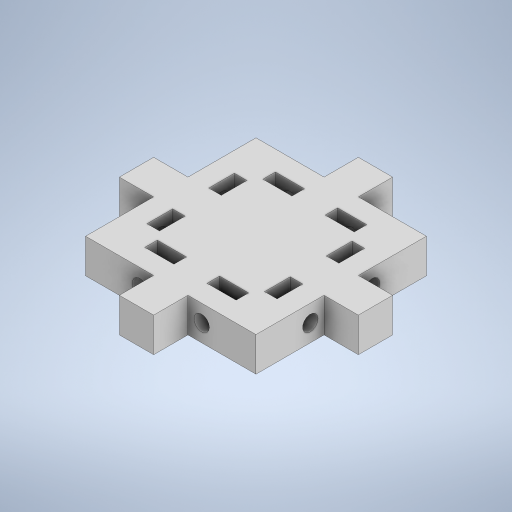
# Autodesk Inventor part: arm_motor_connect
Saved by Autodesk Inventor 2024 (Build 280153000, 153)
## iProperties
Created: 2024-09-18
Part Number: arm_motor_connect
Material: 일반
Document SubType Name: Modeling
Designer: Eungang
Density: 1 g/cm^3
Appearance: 기본값
Author: Eungang
Autodesk Inventor part; units mm, degrees
ref_plane "YZ Plane" through (0, 0, 0) normal (1, 0, 0) x (0, 1, 0)
ref_plane "XZ Plane" through (0, 0, 0) normal (0, 1, 0) x (-1, 0, 0)
sketch "스케치1" plane through (0, 0, 0) normal (0, 0, 1) x (1, 0, 0)
  arc A0 (-4.555, 20.4) -> (-1.5118, 17.2038) centre (-1.355, 20.4) ccw projected
  line L0 (-4.555, 20.4) -> (-4.555, 29.4) projected
  line L1 (-4.555, 29.4) -> (-9.955, 29.4) projected
  line L2 (-9.955, 29.4) -> (-9.955, 17.8) projected
  line L3 (-9.955, 17.8) -> (-4.855, 11.8) projected
  line L4 (-4.855, 11.8) -> (-4.7625, 11.8) projected
  line L5 (-4.7625, 11.8) -> (-4.7625, -3) projected
  line L6 (-4.7625, -3) -> (3.7037, -3) projected
  arc A1 (4.7037, -2) -> (3.7037, -3) centre (4.7037, -3) ccw projected
  line L7 (4.7037, -2) -> (4.7037, 2.1) projected
  arc A2 (5.6987, 3) -> (4.7037, 2.1) centre (4.7037, 3.1) ccw projected
  line L8 (5.6987, 3) -> (9.9088, 3) projected
  arc A3 (10.9037, 2.1) -> (9.9088, 3) centre (10.9037, 3.1) ccw projected
  line L9 (10.9037, 2.1) -> (10.9037, -2) projected
  arc A4 (11.9037, -3) -> (10.9037, -2) centre (10.9037, -3) ccw projected
  line L10 (11.9037, -3) -> (20.4525, -3) projected
  line L11 (20.4525, -3) -> (20.4525, 11.8) projected
  line L12 (20.4525, 11.8) -> (20.545, 11.8) projected
  line L13 (20.545, 11.8) -> (25.645, 17.8) projected
  line L14 (25.645, 17.8) -> (25.645, 29.4) projected
  line L15 (25.645, 29.4) -> (20.245, 29.4) projected
  line L16 (20.245, 29.4) -> (20.245, 20.4) projected
  arc A5 (17.2018, 17.2038) -> (20.245, 20.4) centre (17.045, 20.4) ccw projected
  line L17 (17.2018, 17.2038) -> (-1.5118, 17.2038) projected
  circle A6 centre (13.2469, 0) radius 1.35 projected
  circle A7 centre (2.4432, 0) radius 1.35 projected
  circle A8 centre (18.0506, 0) radius 1.35 projected
  circle A9 centre (-2.3606, 0) radius 1.35 projected
  circle A10 centre (-7.155, 20.9) radius 1.35 projected
  circle A11 centre (-0.655, 14.6) radius 1.35 projected
  circle A12 centre (16.345, 14.6) radius 1.35 projected
  circle A13 centre (22.845, 20.9) radius 1.35 projected
  line L18 (20.4525, -3) -> (-4.855, -3)
  line L19 (-4.855, -3) -> (-4.855, 3)
  line L20 (-4.855, 3) -> (20.4525, 3)
  line L21 (20.4525, 3) -> (20.4525, -3)
  line L22 (22.845, 3) -> (22.845, -11.8) projected
  line L23 (-7.155, 3) -> (-7.155, -11.8) projected
  line L24 (22.745, 3) -> (22.745, -11.8)
  line L25 (-7.055, 3) -> (-7.055, -11.8)
  line L26 (22.745, -3) -> (-7.055, -3)
  line L27 (-7.055, -3) -> (-7.055, 3)
  line L28 (-7.055, 3) -> (22.745, 3)
  line L29 (22.745, 3) -> (22.745, -3)
  point P0 (0, 0)
  point P1 (11.8625, -3)
  point P2 (20.4525, 3)
  point P3 (9.8675, 3)
  point P4 (5.6574, 3)
  point P5 (-4.7625, 3)
  point P6 (3.6625, -3)
  point P7 (-4.855, 3)
  point P8 (-7.055, -3)
  point P9 (-4.855, -3)
  point P10 (-4.7625, -3)
  point P11 (22.745, 1.2049)
  point P12 (20.4525, 3)
  point P13 (20.4525, -3)
  point P14 (11.8987, 3)
  point P15 (3.7037, -3)
  point P16 (11.9037, -3)
  point P17 (5.6987, 3)
  point P18 (3.7088, 3)
  point P19 (5.6987, 3)
  point P20 (11.9037, -3)
  point P21 (-4.7625, 3)
  point P22 (-4.855, -3)
  point P23 (10.9037, -1.792)
  point P24 (-4.7625, -3)
  point P25 (4.7037, -1.792)
  dimension "d7" = 0.1
  dimension "d8" = 0.1
  constraints: 20 end point, 6 parallel, 2 horizontal, 2 perpendicular, 1 point on line
  measures "d7" distance between parallel lines of L22 L24
  measures "d8" distance between parallel lines of L23 L25
extrude "돌출1" add sketch "스케치1" along normal blind 29.8 contours L20 A2 L7 A1 L6 L5 | L5 L18 L19 L20 | L19 L26 L25 L28 | L20 L8 A3 L9 A4 L18 A1 L7 A2 | L28 L24 L26 L11 | L11 L10 A4 L9 A3 L20 | A6 | A7 | A8 | A9
ref_plane "작업 평면4" through (10.8037, 3, 0) normal (0, 1, 0) x (1, 0, 0)
sketch "스케치5" plane through (10.8037, 3, 0) normal (0, 1, 0) x (1, 0, 0)
  line L0 (1.1931, -3.675) -> (1.1931, 6)
  line L1 (3.6931, -3.675) -> (3.6931, 6)
  line L2 (1.1931, -5.675) -> (3.6931, -5.675)
  line L3 (2.4431, 0) -> (2.4431, -3.675)
  line L4 (2.4431, -5.675) -> (2.4431, -4.575)
  line L5 (2.4431, -4.575) -> (2.4431, -3.475)
  line L6 (2.4431, -3.475) -> (-0.1069, -3.475)
  line L7 (2.4431, -3.475) -> (4.9931, -3.475)
  line L8 (4.9931, -3.475) -> (-0.1069, -3.475)
  line L9 (-0.1069, -3.475) -> (-0.1069, -5.675)
  line L10 (-0.1069, -5.675) -> (4.9931, -5.675)
  line L11 (4.9931, -5.675) -> (4.9931, -3.475)
  line L12 (1.1931, -5.675) -> (1.1931, 6)
  line L13 (3.6931, -5.675) -> (3.6931, 6)
  line L14 (1.1931, -5.675) -> (3.6931, -5.675)
  line L15 (2.4431, -3.675) -> (2.4431, -5.675)
  line L16 (-23.9, -14.9) -> (17.9, -14.9)
  line L17 (1.1931, -24.125) -> (3.6931, -24.125)
  line L18 (2.4431, -24.125) -> (2.4431, -25.225)
  line L19 (2.4431, -25.225) -> (2.4431, -26.325)
  line L20 (2.4431, -26.325) -> (-0.1069, -26.325)
  line L21 (2.4431, -26.325) -> (4.9931, -26.325)
  line L22 (4.9931, -26.325) -> (-0.1069, -26.325)
  line L23 (-0.1069, -26.325) -> (-0.1069, -24.125)
  line L24 (-0.1069, -24.125) -> (4.9931, -24.125)
  line L25 (4.9931, -24.125) -> (4.9931, -26.325)
  line L26 (1.1931, -24.125) -> (3.6931, -24.125)
  line L27 (2.4431, -26.125) -> (2.4431, -24.125)
  line L28 (-3, -14.9) -> (-3, -22)
  line L29 (-7.1931, -5.675) -> (-9.6931, -5.675)
  line L30 (-8.4431, -5.675) -> (-8.4431, -4.575)
  line L31 (-8.4431, -4.575) -> (-8.4431, -3.475)
  line L32 (-8.4431, -3.475) -> (-5.8931, -3.475)
  line L33 (-8.4431, -3.475) -> (-10.9931, -3.475)
  line L34 (-10.9931, -3.475) -> (-5.8931, -3.475)
  line L35 (-5.8931, -3.475) -> (-5.8931, -5.675)
  line L36 (-5.8931, -5.675) -> (-10.9931, -5.675)
  line L37 (-10.9931, -5.675) -> (-10.9931, -3.475)
  line L38 (-7.1931, -5.675) -> (-9.6931, -5.675)
  line L39 (-8.4431, -3.675) -> (-8.4431, -5.675)
  line L40 (-7.1931, -24.125) -> (-9.6931, -24.125)
  line L41 (-8.4431, -24.125) -> (-8.4431, -25.225)
  line L42 (-8.4431, -25.225) -> (-8.4431, -26.325)
  line L43 (-7.1931, -24.125) -> (-9.6931, -24.125)
  line L44 (-8.4431, -26.125) -> (-8.4431, -24.125)
  line L45 (-8.4431, -26.325) -> (-10.9931, -26.325)
  line L46 (-10.9931, -24.125) -> (-10.9931, -26.325)
  line L47 (-8.4431, -26.325) -> (-5.8931, -26.325)
  line L48 (-5.8931, -26.325) -> (-5.8931, -24.125)
  line L49 (-10.9931, -26.325) -> (-5.8931, -26.325)
  line L50 (-5.8931, -24.125) -> (-10.9931, -24.125)
  line L51 (-12.1837, -21.5519) -> (-23.8587, -21.5519)
  line L52 (-12.1837, -19.0519) -> (-23.8587, -19.0519)
  line L53 (-12.1837, -19.0519) -> (-12.1837, -21.5519)
  line L54 (-12.1837, -19.0519) -> (-14.3837, -19.0519)
  line L55 (-12.1837, -20.3019) -> (-12.1837, -18.0519)
  line L56 (-12.1837, -20.3019) -> (-12.1837, -22.5519)
  line L57 (-14.3837, -18.0519) -> (-12.1837, -18.0519)
  line L58 (-12.1837, -18.0519) -> (-12.1837, -22.5519)
  line L59 (-12.1837, -22.5519) -> (-14.3837, -22.5519)
  line L60 (-14.3837, -22.5519) -> (-14.3837, -18.0519)
  line L61 (-12.1837, -10.7481) -> (-12.1837, -8.2481)
  line L62 (-12.1837, -10.7481) -> (-14.3837, -10.7481)
  line L63 (-12.1837, -9.4981) -> (-12.1837, -11.7481)
  line L64 (-12.1837, -9.4981) -> (-12.1837, -7.2481)
  line L65 (-14.3837, -11.7481) -> (-12.1837, -11.7481)
  line L66 (-12.1837, -11.7481) -> (-12.1837, -7.2481)
  line L67 (-12.1837, -7.2481) -> (-14.3837, -7.2481)
  line L68 (-14.3837, -7.2481) -> (-14.3837, -11.7481)
  line L69 (6.1837, -19.0519) -> (6.1837, -21.5519)
  line L70 (6.1837, -19.0519) -> (8.3837, -19.0519)
  line L71 (6.1837, -20.3019) -> (6.1837, -18.0519)
  line L72 (6.1837, -20.3019) -> (6.1837, -22.5519)
  line L73 (8.3837, -18.0519) -> (6.1837, -18.0519)
  line L74 (6.1837, -18.0519) -> (6.1837, -22.5519)
  line L75 (6.1837, -22.5519) -> (8.3837, -22.5519)
  line L76 (8.3837, -22.5519) -> (8.3837, -18.0519)
  line L77 (6.1837, -9.4981) -> (6.1837, -7.2481)
  line L78 (6.1837, -7.2481) -> (8.3837, -7.2481)
  line L79 (6.1837, -10.7481) -> (6.1837, -8.2481)
  line L80 (6.1837, -9.4981) -> (6.1837, -11.7481)
  line L81 (6.1837, -10.7481) -> (8.3837, -10.7481)
  line L82 (8.3837, -11.7481) -> (6.1837, -11.7481)
  line L83 (8.3837, -7.2481) -> (8.3837, -11.7481)
  line L84 (6.1837, -11.7481) -> (6.1837, -7.2481)
  point P0 (-0.1069, -3.475)
  point P1 (1.1931, -26.125)
  point P2 (3.6931, -26.125)
  point P3 (-7.1931, -3.675)
  point P4 (-9.6931, -3.675)
  point P5 (-7.1931, -26.125)
  point P6 (-9.6931, -26.125)
  point P7 (-0.1069, -26.325)
  point P8 (3.6931, -24.125)
  point P9 (1.1931, -24.125)
  dimension "d24" = 1.1
  dimension "d25" = 1.1
  dimension "d26" = 2.55
  dimension "d27" = 2.55
  dimension "d28" = 2.2
  dimension "d29" = 2.25
  dimension "d30" = 2.25
  constraints: 170 end point, 78 symmetric about line, 7 vertical, 5 horizontal, 5 perpendicular, 5 point on line, 4 midpoint, 4 parallel, 8 other
  measures "d24" distance of L4.start L4.end
  measures "d25" distance of L4.end L5.end
  measures "d26" distance of L5.end L6.end
  measures "d27" distance of L5.end L7.end
  measures "d28" distance of L52.start L54.end
  measures "d29" distance of L55.start L55.end
  measures "d30" distance of L55.start L56.end
extrude "돌출4" cut sketch "스케치5" against normal blind 6
sketch "스케치6" plane through (-7.055, -3, 29.8) normal (-1, 0, 0) x (0, 0, 1)
  circle A0 centre (-9.4981, 3) radius 1.35 projected
  circle A1 centre (-20.3019, 3) radius 1.35 projected
  point P0 (-29.8, 3)
extrude "돌출5" cut sketch "스케치6" against normal up to next
sketch "스케치7" plane through (0, 0, 0) normal (0, 0, -1) x (-1, 0, 0)
  circle A0 centre (-13.2469, 0) radius 1.35 projected
  circle A1 centre (-2.4432, 0) radius 1.35 projected
  point P0 (0, 0)
extrude "돌출6" cut sketch "스케치7" against normal up to next
sketch "스케치8" plane through (22.745, -3, 0) normal (1, 0, 0) x (0, 0, -1)
  circle A0 centre (-20.3019, 3) radius 1.35 projected
  circle A1 centre (-9.4981, 3) radius 1.35 projected
  point P0 (0, 3)
extrude "돌출7" cut sketch "스케치8" against normal up to next
sketch "스케치9" plane through (0, 0, 29.8) normal (0, 0, 1) x (1, 0, 0)
  circle A0 centre (2.4432, 0) radius 1.35 projected
  circle A1 centre (13.2469, 0) radius 1.35 projected
  point P0 (0, 0)
extrude "돌출8" cut sketch "스케치9" against normal up to next
sketch "스케치10" plane through (-7.055, 3, 0) normal (0, 1, 0) x (1, 0, 0)
  line L0 (24.0424, -18.0519) -> (26.2424, -18.0519) projected
  line L1 (26.2424, -18.0519) -> (26.2424, -22.5519) projected
  line L2 (26.2424, -22.5519) -> (24.0424, -22.5519) projected
  line L3 (24.0424, -22.5519) -> (24.0424, -18.0519) projected
  line L4 (11.9656, -3.475) -> (11.9656, -5.675) projected
  line L5 (11.9656, -5.675) -> (6.8656, -5.675) projected
  line L6 (6.8656, -5.675) -> (6.8656, -3.475) projected
  line L7 (6.8656, -3.475) -> (11.9656, -3.475) projected
  line L8 (11.9656, -24.125) -> (11.9656, -26.325) projected
  line L9 (11.9656, -26.325) -> (6.8656, -26.325) projected
  line L10 (6.8656, -26.325) -> (6.8656, -24.125) projected
  line L11 (6.8656, -24.125) -> (11.9656, -24.125) projected
  line L12 (3.475, -7.2481) -> (5.675, -7.2481) projected
  line L13 (5.675, -7.2481) -> (5.675, -11.7481) projected
  line L14 (5.675, -11.7481) -> (3.475, -11.7481) projected
  line L15 (3.475, -11.7481) -> (3.475, -7.2481) projected
  line L16 (26.2424, -11.7481) -> (24.0424, -11.7481) projected
  line L17 (24.0424, -11.7481) -> (24.0424, -7.2481) projected
  line L18 (24.0424, -7.2481) -> (26.2424, -7.2481) projected
  line L19 (26.2424, -7.2481) -> (26.2424, -11.7481) projected
  line L20 (22.8519, -3.475) -> (22.8519, -5.675) projected
  line L21 (22.8519, -5.675) -> (17.7519, -5.675) projected
  line L22 (17.7519, -5.675) -> (17.7519, -3.475) projected
  line L23 (17.7519, -3.475) -> (22.8519, -3.475) projected
  line L24 (22.8519, -24.125) -> (22.8519, -26.325) projected
  line L25 (22.8519, -26.325) -> (17.7519, -26.325) projected
  line L26 (17.7519, -26.325) -> (17.7519, -24.125) projected
  line L27 (17.7519, -24.125) -> (22.8519, -24.125) projected
  line L28 (3.475, -18.0519) -> (5.675, -18.0519) projected
  line L29 (5.675, -18.0519) -> (5.675, -22.5519) projected
  line L30 (5.675, -22.5519) -> (3.475, -22.5519) projected
  line L31 (3.475, -22.5519) -> (3.475, -18.0519) projected
  line L32 (29.8, 0) -> (0, 0) projected
  line L33 (0, 0) -> (0, -29.8) projected
  line L34 (29.8, -29.8) -> (0, -29.8) projected
  line L35 (29.8, 0) -> (29.8, -29.8) projected
  line L36 (0, -14.9) -> (-6, -14.9)
  line L37 (-6, -14.9) -> (-6, -11.9)
  line L38 (-6, -11.9) -> (0, -11.9)
  line L39 (0, -11.9) -> (0, -17.9)
  line L40 (0, -17.9) -> (-6, -17.9)
  line L41 (-6, -17.9) -> (-6, -11.9)
  line L42 (14.9, 0) -> (14.9, -2)
  line L43 (29.8, -14.9) -> (35.8, -14.9)
  line L44 (35.8, -14.9) -> (35.8, -11.9)
  line L45 (35.8, -11.9) -> (29.8, -11.9)
  line L46 (29.8, -11.9) -> (29.8, -17.9)
  line L47 (29.8, -17.9) -> (35.8, -17.9)
  line L48 (35.8, -17.9) -> (35.8, -11.9)
  line L49 (14.9, 0) -> (14.9, 3)
  line L50 (14.9, 3) -> (14.9, 6)
  line L51 (14.9, 6) -> (11.9, 6)
  line L52 (11.9, 6) -> (17.9, 6)
  line L53 (17.9, 6) -> (17.9, 0)
  line L54 (17.9, 0) -> (11.9, 0)
  line L55 (11.9, 0) -> (11.9, 6)
  line L56 (14.9, -29.8) -> (14.9, -32.8)
  line L57 (14.9, -32.8) -> (14.9, -35.8)
  line L58 (14.9, -35.8) -> (11.9, -35.8)
  line L59 (11.9, -35.8) -> (17.9, -35.8)
  line L60 (17.9, -35.8) -> (17.9, -29.8)
  line L61 (17.9, -29.8) -> (11.9, -29.8)
  line L62 (11.9, -29.8) -> (11.9, -35.8)
  point P0 (7.055, 0)
  point P1 (0, -11.9)
  dimension "d39" = 3
  dimension "d40" = 6
  dimension "d41" = 3
  dimension "d42" = 6
  constraints: 54 end point, 13 symmetric about line, 4 parallel, 4 perpendicular, 4 point on line, 3 horizontal, 2 midpoint, 2 vertical
  measures "d39" distance of L36.end L37.end
  measures "d40" distance of L38.end L39.end
  measures "d41" distance of L50.end L51.end
  measures "d42" distance of L53.end L54.end
extrude "돌출9" add sketch "스케치10" against normal blind 6 contours L32 L49 L50 L52 L53 | L45 L44 L43 L35 | L32 L55 L51 L50 L49 | L43 L48 L47 L35 | L33 L36 L37 L38 | L60 L59 L57 L56 L34 | L33 L40 L41 L36 | L56 L57 L58 L62 L34
